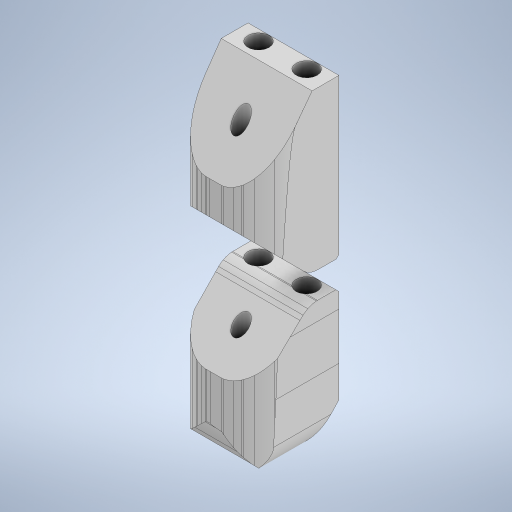
# Autodesk Inventor part: Finger_Thumb
Saved by Autodesk Inventor 2024 (Build 280153000, 153)
## iProperties
Created: 2025-05-19
Part Number: Finger_Thumb
Material: Generic
Document SubType Name: Modeling
Designer: Mehdi Charfeddine
Density: 1 g/cm^3
Appearance: Default
Author: Mehdi Charfeddine
Autodesk Inventor part; units mm, degrees
ref_plane "YZ Plane" through (0, 0, 0) normal (1, 0, 0) x (0, 1, 0)
ref_plane "XZ Plane" through (0, 0, 0) normal (0, 1, 0) x (-1, 0, 0)
ref_plane "XY Plane" through (0, 0, 0) normal (0, 0, 1) x (1, 0, 0)
sketch "Sketch1" plane through (0, 0, 0) normal (0, 1, 0) x (-1, 0, 0)
  line L0 (-3746.0785, 0) -> (-3771.9, 25.4)
  line L1 (-3771.9, 25.4) -> (-3771.9, 152.4147)
  line L2 (-3771.9, 152.4147) -> (-3770.1202, 229.6232)
  line L3 (-3770.1202, 229.6232) -> (-3341.8766, 229.6232)
  line L4 (-3341.8766, 229.6232) -> (-3340.0962, 152.4148)
  line L5 (-3340.0962, 152.4148) -> (-3340.0962, 25.4)
  line L6 (-3340.0962, 25.4) -> (-3365.9269, 0)
  line L7 (-3365.9269, 0) -> (-3746.0785, 0)
  arc A0 (-3750.1396, 308.4294) -> (-3770.1202, 229.6232) centre (-3588.1759, 225.4289) ccw
  arc A1 (-3706.5456, 362.7383) -> (-3750.1396, 308.4294) centre (-3581.9198, 218.0497) ccw
  arc A2 (-3676.9276, 383.4396) -> (-3706.5456, 362.7383) centre (-3576.8538, 208.7227) ccw
  arc A3 (-3671.2815, 386.4607) -> (-3676.9276, 383.4396) centre (-3576.7378, 202.982) ccw
  arc A4 (-3645.0163, 397.4436) -> (-3671.2815, 386.4607) centre (-3579.4325, 203.7052) ccw
  arc A5 (-3605.9928, 405.6246) -> (-3645.0163, 397.4436) centre (-3588.7852, 226.3822) ccw
  arc A6 (-3596.5817, 406.2386) -> (-3605.9928, 405.6246) centre (-3591.3752, 253.9874) ccw
  arc A7 (-3596.5817, 406.2386) -> (-3535.9827, 406.4267) centre (-3632.6291, 21775.8796) ccw
  arc A8 (-3518.8941, 406.3471) -> (-3535.9827, 406.4267) centre (-3530.6798, -289.9638) ccw
  arc A9 (-3497.9469, 404.6463) -> (-3518.8941, 406.3471) centre (-3523.3838, 221.2122) ccw
  arc A10 (-3475.9118, 400.1146) -> (-3497.9469, 404.6463) centre (-3524.5859, 219.2789) ccw
  arc A11 (-3465.1413, 396.8147) -> (-3475.9118, 400.1146) centre (-3518.1143, 243.1426) ccw
  arc A12 (-3430.836, 380.9858) -> (-3465.1413, 396.8147) centre (-3524.5716, 222.9256) ccw
  arc A13 (-3389.6227, 347.4514) -> (-3430.836, 380.9858) centre (-3517.1244, 232.8461) ccw
  arc A14 (-3354.8151, 292.1906) -> (-3389.6227, 347.4514) centre (-3519.2794, 227.1908) ccw
  arc A15 (-3343.6124, 250.4134) -> (-3354.8151, 292.1906) centre (-3519.7432, 225.5735) ccw
  arc A16 (-3341.8766, 229.6232) -> (-3343.6124, 250.4134) centre (-3521.9514, 225.0563) ccw
  arc A17 (-3721.0925, 76.4394) -> (-3698.1313, 33.7101) centre (-3670.0254, 76.3471) ccw
  circle A18 centre (-3670.0254, 76.3471) radius 50
  circle A19 centre (-3441.0009, 76.3471) radius 50
  point P0 (0, 0)
  dimension "d0" = 100
  dimension "d1" = 100
  constraints: 36 point on circle, 20 centre point, 16 end point, 2 perpendicular, 1 coincident, 1 tangent, 1 vertical
  measures "d0" diameter of A18
  measures "d1" diameter of A19
extrude "Extrusion1" add sketch "Sketch1" along normal blind 3000
sketch "Sketch2" plane through (0, 0, 0) normal (1, 0, 0) x (0, 1, 0)
  line L0 (2044.6604, 152.439) -> (2044.6604, 25.012)
  line L1 (2044.6604, 25.012) -> (2018.5463, 0)
  line L2 (2018.5463, 0) -> (1308.0626, 0)
  line L3 (1308.0626, 0) -> (1282.7423, 25.425)
  line L4 (1282.7423, 25.425) -> (1282.7423, 112.0884)
  arc A0 (1293.6006, 156.6793) -> (1282.7423, 112.0884) centre (1385.9607, 110.5712) ccw
  arc A1 (1311.8264, 181.4695) -> (1293.6006, 156.6793) centre (1391.2484, 103.9832) ccw
  line L5 (1311.8264, 181.4695) -> (1536.7024, 406.4179)
  line L6 (1536.7024, 406.4179) -> (1694.1598, 406.4179)
  line L7 (1694.1598, 406.4179) -> (2044.6604, 152.439)
  line L8 (1155.8322, 25.425) -> (1130.4154, 0)
  line L9 (1130.4154, 0) -> (689.571, 0)
  line L10 (689.571, 0) -> (520.6979, 152.4025)
  line L11 (520.6979, 152.4025) -> (520.6979, 229.6018)
  line L12 (520.6979, 229.6018) -> (520.6979, 239.4411)
  arc A2 (521.1873, 250.9055) -> (520.6979, 239.4411) centre (763.1004, 234.8361) ccw
  arc A3 (546.0871, 327.2338) -> (521.1873, 250.9055) centre (688.2516, 238.6313) ccw
  arc A4 (581.5525, 367.8542) -> (546.0871, 327.2338) centre (688.5204, 238.6688) ccw
  arc A5 (623.2992, 393.1802) -> (581.5525, 367.8542) centre (689.7234, 236.6182) ccw
  arc A6 (662.2216, 404.3171) -> (623.2992, 393.1802) centre (688.4624, 239.0248) ccw
  arc A7 (683.0136, 406.2983) -> (662.2216, 404.3171) centre (688.4624, 239.0248) ccw
  arc A8 (688.4021, 406.4009) -> (683.0136, 406.2983) centre (688.7576, 246.1487) ccw
  line L13 (688.4021, 406.4009) -> (901.6882, 406.4009)
  line L14 (901.6882, 406.4009) -> (1113.4921, 194.5352)
  line L15 (1113.4921, 194.5352) -> (1127.9026, 180.0918)
  line L16 (1127.9026, 180.0918) -> (1128.7816, 180.8543)
  arc A9 (1143.7208, 158.1069) -> (1127.9026, 180.0918) centre (1056.4195, 111.9766) ccw
  arc A10 (1155.5794, 117.7762) -> (1143.7208, 158.1069) centre (1053.9046, 109.7891) ccw
  arc A11 (1155.5794, 117.7762) -> (1155.8322, 103.9832) centre (17018.1258, 401.6638) ccw
  line L17 (1155.8322, 103.9832) -> (1155.8322, 25.425)
  line L18 (4921.342, 1654.0698) -> (-2748.1755, 1654.0698)
  line L19 (-2748.1755, 1654.0698) -> (-2748.1755, -1427.7454)
  line L20 (-2748.1755, -1427.7454) -> (4921.342, -1427.7454)
  line L21 (4921.342, -1427.7454) -> (4921.342, 1654.0698)
  point P0 (0, 0)
  constraints: 44 end point, 26 point on circle, 12 centre point, 4 parallel, 3 horizontal, 3 perpendicular, 3 point on line, 2 vertical, 1 concentric
sketch "Sketch3" plane through (0, 0, 0) normal (0, 0, 1) x (1, 0, 0)
  line L0 (3748.2421, 645.64) -> (3752.0678, 840.2646)
  line L1 (3752.0678, 840.2646) -> (3755.3768, 1066.9304)
  line L2 (3755.3768, 1066.9304) -> (3757.0985, 1155.6727)
  line L3 (3757.0985, 1155.6727) -> (3354.8296, 1155.6727)
  line L4 (3354.8296, 1155.6727) -> (3356.2277, 1071.8651)
  line L5 (3356.2277, 1071.8651) -> (3357.9282, 969.9368)
  line L6 (3357.9282, 969.9368) -> (3359.4188, 880.5862)
  line L7 (3359.4188, 880.5862) -> (3361.1562, 776.4444)
  line L8 (3361.1562, 776.4444) -> (3363.3385, 645.6358)
  arc A0 (3363.3385, 645.6358) -> (3491.3103, 520.7049) centre (3490.1595, 647.5349) ccw
  line L9 (3751.2288, 797.5807) -> (3748.2421, 645.64)
  arc A1 (3620.1063, 520.7049) -> (3748.2421, 645.64) centre (3622.1983, 646.7362) ccw
  line L10 (3620.1063, 520.7049) -> (3491.3103, 520.7049)
  line L11 (3759.2012, 1282.6994) -> (3352.8001, 1282.7)
  line L12 (3352.8001, 1282.7) -> (3340.1001, 2044.7)
  line L13 (3340.1001, 2044.7) -> (3771.9003, 2044.7)
  line L14 (3771.9003, 2044.7) -> (3759.2012, 1282.6994)
  line L15 (4080.489, 275.1554) -> (3053.9865, 275.1554)
  line L16 (3053.9865, 275.1554) -> (3053.9865, 2241.796)
  line L17 (3053.9865, 2241.796) -> (4080.489, 2241.796)
  line L18 (4080.489, 2241.796) -> (4080.489, 275.1554)
  point P0 (0, 0)
  constraints: 38 end point, 5 point on line, 4 horizontal, 4 point on circle, 2 centre point, 2 parallel, 1 collinear, 1 perpendicular
sketch "Sketch4" plane through (0, 0, 0) normal (0, 1, 0) x (-1, 0, 0)
  circle A0 centre (-3555.3066, 273.225) radius 35
  point P0 (0, 0)
  dimension "d4" = 70
  constraints: 1 centre point
  measures "d4" diameter of A0
extrude "Extrusion2" cut sketch "Sketch2" along normal mid plane 30000
extrude "Extrusion3" cut sketch "Sketch3" along normal mid plane 30000
extrude "Extrusion4" cut sketch "Sketch4" along normal blind 30000
body "Solid1"
